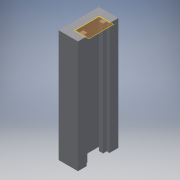
# Autodesk Inventor part: Right Gun Mount
Saved by Autodesk Inventor 2018 (Build 220112000, 112)
## iProperties
Created: 2018-11-09
Part Number: Right Gun Mount
Material: Generic
Document SubType Name: Modeling
Designer: Cameron
Mass: 117.856 g
Surface Area: 263.862 cm^2
Volume: 117.856 cm^3
Density: 1 g/cm^3
Appearance: Default
Author: Cameron
Autodesk Inventor part; units mm, degrees
ref_plane "YZ Plane" through (0, 0, 0) normal (1, 0, 0) x (0, 1, 0)
ref_plane "XZ Plane" through (0, 0, 0) normal (0, 1, 0) x (-1, 0, 0)
ref_plane "XY Plane" through (0, 0, 0) normal (0, 0, 1) x (1, 0, 0)
ref_plane "Work Plane1" through (0, 0, 0) normal (0, 0, 1) x (1, 0, 0)
sketch "Sketch2" plane through (0, 0, 0) normal (0, 0, 1) x (1, 0, 0)
  line L0 (-17.5, 25.27) -> (-2, 25.27)
  line L1 (-2, 25.27) -> (-2, -7)
  line L2 (-2, -7) -> (-17.5, -7)
  line L3 (-17.5, -7) -> (-17.5, 25.27)
  line L4 (-4.25, 18.27) -> (-4.25, 15.385) projected
  line L5 (-4.25, 15.385) -> (-7.65, 15.385) projected
  line L6 (-7.65, 15.385) -> (-7.65, 18.27) projected
  line L7 (-7.65, 18.27) -> (-10.5, 18.27) projected
  line L8 (-10.5, 0) -> (-10.5, 18.27) projected
  line L9 (-7.65, 0) -> (-10.5, 0) projected
  line L10 (-7.65, 0) -> (-7.65, 2.885) projected
  line L11 (-7.65, 2.885) -> (-4.25, 2.885) projected
  line L12 (-4.25, 2.885) -> (-4.25, 0) projected
  line L13 (0, 0) -> (-4.25, 0) projected
  line L14 (0, 18.27) -> (0, 0) projected
  line L15 (0, 18.27) -> (-4.25, 18.27) projected
  dimension "d6" = 2
  dimension "d7" = 7
  dimension "d9" = 7
  dimension "d10" = 7
  constraints: 8 end point, 2 parallel, 1 horizontal, 1 perpendicular
  measures "d6" distance between parallel lines of L14 L1
  measures "d7" distance between parallel lines of L9 L2
  measures "d9" distance between parallel lines of L0 L15
  measures "d10" distance between parallel lines of L3 L8
extrude "Extrusion2" add sketch "Sketch2" against normal blind 90 contours L0 L1 L15 L4 L5 L6 L7 L8 L9 L10 L11 L12 L13 L2 L3 | L1 L13 L12 L11 L10 L9 L8 L7 L6 L5 L4 L15
ref_plane "Work Plane2" through (0, 0, 0) normal (0, 0, 1) x (1, 0, 0)
sketch "Sketch3" plane through (0, 0, 0) normal (0, 0, 1) x (1, 0, 0)
  line L0 (-4.25, 18.27) -> (-4.25, 15.385) projected
  line L1 (-4.25, 15.385) -> (-7.65, 15.385) projected
  line L2 (-7.65, 15.385) -> (-7.65, 18.27) projected
  line L3 (-7.65, 18.27) -> (-10.5, 18.27) projected
  line L4 (-10.5, 0) -> (-10.5, 18.27) projected
  line L5 (-7.65, 0) -> (-10.5, 0) projected
  line L6 (-7.65, 0) -> (-7.65, 2.885) projected
  line L7 (-7.65, 2.885) -> (-4.25, 2.885) projected
  line L8 (-4.25, 2.885) -> (-4.25, 0) projected
  line L9 (0, 0) -> (-4.25, 0) projected
  line L10 (0, 18.27) -> (0, 0) projected
  line L11 (0, 18.27) -> (-4.25, 18.27) projected
extrude "Extrusion3" cut sketch "Sketch3" against normal blind 90
sketch "Sketch4" plane through (-17.5, -7, 0) normal (0, -1, 0) x (1, 0, 0)
  line L0 (15.5, 0) -> (0, 0) projected
  line L1 (0, 0) -> (0, -90) projected
  line L2 (15.5, -90) -> (0, -90) projected
  line L3 (15.5, 0) -> (15.5, -90) projected
  line L4 (0, 0) -> (0, -90) projected
  line L5 (0, -90) -> (15.5, -90) projected
  line L6 (0, 0) -> (13.5, 0)
  line L7 (13.5, 0) -> (13.5, -90)
  line L8 (13.5, -90) -> (0, -90)
  line L9 (0, -90) -> (0, 0)
  point P0 (17.5, 0)
  dimension "d15" = 2
  constraints: 8 end point, 2 parallel, 1 horizontal, 1 perpendicular, 1 point on line
  measures "d15" distance between parallel lines of L3 L7
extrude "Extrusion4" add sketch "Sketch4" along normal blind 70 contours L7 L2 L1 L0
sketch "Sketch5" plane through (-17.5, 25.27, -90) normal (-1, 0, 0) x (0, 0, 1)
  circle A0 centre (42.6, -48) radius 18 projected
  arc A1 (13.1658, -6.85) -> (11.1891, -8.5459) centre (13.1658, -8.85) ccw projected
  line L0 (11.1891, -8.5459) -> (-28.55, -266.85) projected
  line L1 (-28.55, -266.85) -> (113.75, -266.85) projected
  line L2 (113.75, -266.85) -> (74.0109, -8.5459) projected
  arc A2 (74.0109, -8.5459) -> (72.0342, -6.85) centre (72.0342, -8.85) ccw projected
  line L3 (72.0342, -6.85) -> (13.1658, -6.85) projected
  line L4 (90, 0) -> (90, -102.27) projected
  line L5 (90, 0) -> (0, 0) projected
  line L6 (0, 0) -> (0, -102.27) projected
  line L7 (90, -102.27) -> (0, -102.27) projected
  line L8 (90, -102.27) -> (113.75, -266.85)
  line L9 (90, -102.27) -> (0, -102.27) projected
  line L10 (0, -102.27) -> (90, -102.27)
  line L11 (90, -102.27) -> (113.75, -266.85)
  line L12 (0, -102.27) -> (-28.55, -266.85)
  line L13 (-28.55, -266.85) -> (113.75, -266.85)
  line L14 (113.75, -266.85) -> (90, -102.27)
  point P0 (90, -25.27)
  dimension "d18" = 164.58
  constraints: 12 end point, 3 collinear
  measures "d18" vertical distance of L4.end L8.end
extrude "Extrusion5" add sketch "Sketch5" against normal blind 13.7 contours L12 L7 L2 L1 | L7 L8 L2
body "Solid2"
